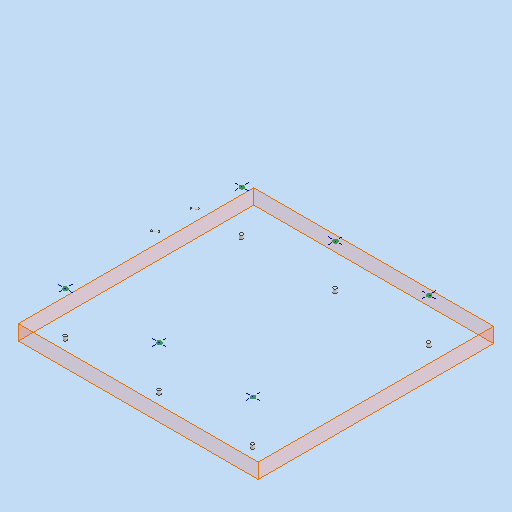
# Autodesk Inventor part: HF-Kabelführung-V3-XGantry-LängenSkizze
Saved by Autodesk Inventor 2023.2 (Build 272271000, 271)
## iProperties
Created: 2023-12-13
Part Number: HF-Kabelführung-V3-XGantry-LängenSkizze
Material: Generisch
Document SubType Name: Modeling
Designer: Nils Bade
Density: 1 g/cm^3
Appearance: Vorgabe
Auf Bestellliste: True
Author: Nils Bade
Autodesk Inventor part; units mm, degrees
ref_plane "YZ Plane" through (0, 0, 0) normal (1, 0, 0) x (0, 1, 0)
ref_plane "XY Plane" through (0, 0, 0) normal (0, 0, 1) x (1, 0, 0)
sketch "S-Orientierung" plane through (0, 0, 0) normal (0, 1, 0) x (-1, 0, 0)
  line L0 (290.75, 0) -> (-290.75, 0)
  line L1 (-290.75, 0) -> (-290.75, -564.4)
  line L2 (-290.75, -564.4) -> (290.75, -564.4)
  line L3 (290.75, -564.4) -> (290.75, 0)
  line L4 (0, -718.1) -> (0, 161.1) construction
  line L5 (-448, 0) -> (448, 0) construction
  line L6 (320, 35.5) -> (-320, 35.5)
  line L7 (-320, 35.5) -> (-320, -592.5)
  line L8 (-320, -592.5) -> (320, -592.5)
  line L9 (320, -592.5) -> (320, 35.5)
  point P0 (0, 0)
  point P1 (0, -19.5)
  point P2 (0, -124.5)
  dimension "d2" = 640
  dimension "d3" = 628
  dimension "d4" = 35.5
  dimension "d67" = 55
  dimension "d87" = 29.25
  dimension "d88" = 28.1
  dimension "d89" = 564.4
  dimension "d90" = 581.5
  dimension "d105" = 160
  constraints: 16 end point, 4 parallel, 2 horizontal, 2 perpendicular, 2 point on line, 1 collinear, 2 other
  measures "d2" distance of L6.start L6.end
  measures "d3" distance of L6.end L7.end
  measures "d4" distance between parallel lines of L6 L0
  measures "d67" distance from line of L6 point (0, -19.5)
  measures "d87" distance between parallel lines of L9 L3
  measures "d88" distance between parallel lines of L8 L2
  measures "d89" distance between parallel lines of L0 L2
  measures "d90" distance between parallel lines of L1 L3
  measures "d105" distance from line of L6 point (0, -124.5)
surface extrude "Ex-Innenseiten-4040-Profile" sketch "S-Orientierung" along normal mid plane 40 shown yes curves L6 L7 L8 L9
ref_plane "Deckenebene" through (0, 365.5, 0) normal (0, 1, 0) x (-1, 0, 0)
sketch "HF-Anschlusspunkte" plane through (0, 0, 0) normal (0, 1, 0) x (-1, 0, 0)
  line L0 (40, -12) -> (-40, -12)
  line L1 (-40, -12) -> (-40, -93.7)
  line L2 (-40, -93.7) -> (40, -93.7)
  line L3 (40, -93.7) -> (40, -12)
  line L4 (-25, -12) -> (-25, -93.7) construction
  line L5 (25, -93.7) -> (25, -12) construction
  circle A0 centre (0, -19.5) radius 4.5
  line L6 (320, 35.5) -> (-320, 35.5) construction
  line L7 (0, -718.1) -> (0, 161.1) projected
  line L8 (40, -482) -> (-40, -482)
  line L9 (-40, -482) -> (-40, -563.7)
  line L10 (-40, -563.7) -> (40, -563.7)
  line L11 (40, -563.7) -> (40, -482)
  line L12 (-25, -482) -> (-25, -563.7) construction
  line L13 (25, -563.7) -> (25, -482) construction
  circle A1 centre (0, -489.5) radius 4.5
  line L14 (-320, -592.5) -> (320, -592.5) projected
  line L15 (296.8699, -564.4) -> (-360.8589, -564.4) construction
  line L16 (-290.75, -592.5) -> (-290.75, 35.5) construction
  line L17 (-320, 35.5) -> (-320, -592.5) construction
  line L18 (-210, -482) -> (-290, -482)
  circle A2 centre (-250, -489.5) radius 4.5
  line L19 (-275, -482) -> (-275, -563.7) construction
  line L20 (-290, -482) -> (-290, -563.7)
  line L21 (-210, -563.7) -> (-210, -482)
  line L22 (-290, -563.7) -> (-210, -563.7)
  line L23 (-225, -563.7) -> (-225, -482) construction
  line L24 (-225, -93.7) -> (-225, -12) construction
  line L25 (-210, -93.7) -> (-210, -12)
  line L26 (-210, -12) -> (-290, -12)
  line L27 (-290, -93.7) -> (-210, -93.7)
  circle A3 centre (-250, -19.5) radius 4.5
  line L28 (-275, -12) -> (-275, -93.7) construction
  line L29 (-290, -12) -> (-290, -93.7)
  line L30 (210, -482) -> (290, -482)
  circle A4 centre (250, -489.5) radius 4.5
  line L31 (275, -482) -> (275, -563.7) construction
  line L32 (290, -482) -> (290, -563.7)
  line L33 (210, -563.7) -> (210, -482)
  line L34 (290, -563.7) -> (210, -563.7)
  line L35 (225, -563.7) -> (225, -482) construction
  line L36 (225, -93.7) -> (225, -12) construction
  line L37 (210, -93.7) -> (210, -12)
  line L38 (210, -12) -> (290, -12)
  line L39 (290, -93.7) -> (210, -93.7)
  circle A5 centre (250, -19.5) radius 4.5
  line L40 (275, -12) -> (275, -93.7) construction
  line L41 (290, -12) -> (290, -93.7)
  line L42 (290.75, -592.5) -> (290.75, 35.5) construction
  point P0 (0, 0)
  point P1 (0, -93.7)
  point P2 (0, -470)
  point P3 (0, -563.7)
  point P4 (-250, -470)
  point P5 (-250, -563.7)
  point P6 (-250, -93.7)
  point P7 (-250, 0)
  point P8 (250, -470)
  point P9 (250, -563.7)
  point P10 (250, -93.7)
  point P11 (250, 0)
  point P12 (40, -522.85)
  point P13 (40, -52.85)
  point P14 (-250, -482)
  dimension "d68" = 80
  dimension "d69" = 81.7
  dimension "d70" = 15
  dimension "d71" = 15
  dimension "d72" = 40
  dimension "d73" = 7.5
  dimension "d74" = 9
  dimension "d75" = 47.5
  dimension "d79" = 470
  dimension "d84" = 28.8
  dimension "d85" = 28.1
  dimension "d86" = 29.25
  dimension "d93" = 250
  dimension "d98" = 470
  dimension "d99" = 500
  dimension "d109" = 55
  constraints: 78 end point, 27 point on line, 24 symmetric about line, 6 centre point, 4 midpoint, 4 perpendicular, 3 horizontal, 2 parallel, 1 collinear, 1 vertical, 55 other
  measures "d68" distance between parallel lines of L1 L3
  measures "d69" distance between parallel lines of L2 L0
  measures "d70" distance between parallel lines of L1 L4
  measures "d71" distance between parallel lines of L3 L5
  measures "d72" distance from line of L1 A0.centre
  measures "d73" distance from line of L0 A0.centre
  measures "d74" diameter of A0
  measures "d75" distance between parallel lines of L6 L0
  measures "d79" distance of point (0, 0) point (0, -470)
  measures "d84" distance between parallel lines of L14 L10
  measures "d85" distance between parallel lines of L14 L15
  measures "d86" distance between parallel lines of L17 L16
  measures "d93" distance of point (0, -470) point (-250, -470)
  measures "d98" distance of point (40, -522.85) point (40, -52.85)
  measures "d99" horizontal distance of point (250, -470) point (-250, -482)
  measures "d109" distance from line of L6 A0.centre
ref_plane "KnickHöhe-HF-Kabel" through (0, 109, 0) normal (0, 1, 0) x (-1, 0, 0)
extrude "Ex-HF-Probeanschlüsse" add sketch "HF-Anschlusspunkte" against normal blind 10 contours L7 A0 | A0 L7 | A1 L7 | L7 A1 | A2 | A3 | A4 | A5
sketch "S-HF-Kabeleinlass" plane through (0, 0, 0) normal (1, 0, 0) x (0, 1, 0)
  line L0 (-75.3867, -19.5) -> (452.3202, -19.5) projected
  line L1 (365.5, 100.2641) -> (365.5, -592.4607) projected
  line L2 (365.5, -19.5) -> (365.5, -19.5) construction
  line L3 (365.5, -19.5) -> (376.9335, 0.3034)
  line L4 (365.5, -19.5) -> (363.7679, -18.5)
  line L5 (363.7679, -18.5) -> (375.2015, 1.3034)
  line L6 (375.2015, 1.3034) -> (376.9335, 0.3034)
  point P0 (0, 0)
  dimension "d102" = 30
  dimension "d104" = 2
  constraints: 10 end point, 3 perpendicular, 3 point on line
  measures "d102" angle of L1 L3
  measures "d104" distance of L5.end L3.end
revolve "Um-HF-Kabeleinlass" add sketch "S-HF-Kabeleinlass" angle 360 about axis through (0, 365.5, -19.5) along (0, 0.5, 0.8660254) separate body
sketch "S-KabelKnickPunkte" plane through (0, 109, 0) normal (0, 1, 0) x (-1, 0, 0)
  circle A0 centre (0, -19.5) radius 4.5 projected
  circle A1 centre (-250, -19.5) radius 4.5 projected
  circle A2 centre (-250, -489.5) radius 4.5 projected
  circle A3 centre (0, -489.5) radius 4.5 projected
  circle A4 centre (250, -489.5) radius 4.5 projected
  circle A5 centre (250, -19.5) radius 4.5 projected
  constraints: 6 coincident
pattern_linear "Rechteckige Anordnung3" count 2 spacing 105 along (0, 0, -1) bodies 2
equation "\"d71\" = d70"
